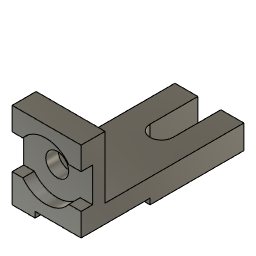
Tutorial Part 12 v5 (Autodesk Fusion 360 design; units mm, degrees)
Autodesk Fusion 360 part; units mm, degrees
sketch "Sketch1" plane through (0, 0, 0) normal (0, 1, 0) x (1, 0, 0)
  line L0 (-35.1053, -42) -> (36.8947, -42)
  line L1 (36.8947, -42) -> (36.8947, 48)
  line L2 (36.8947, 48) -> (-35.1053, 48)
  line L3 (-35.1053, 48) -> (-35.1053, -42)
  point P0 (0.8947, 48)
  dimension "d3" = 90
  dimension "d4" = 72
  dimension "d7" = 48
  constraint horizontal L0
  constraint vertical L1
  constraint horizontal L2
  constraint vertical L3
  constraint midpoint L2 P0
  measures "d3" distance of L0.start L2.end
  measures "d4" distance of L1.end L2.end
  measures "d7" vertical distance of origin P0
extrude "Extrude1" add sketch "Sketch1" along normal blind 25
sketch "Sketch2" plane through (0, 0, 0) normal (0, -1, 0) x (1, 0, 0)
  line L0 (-35.1053, 42) -> (-35.1053, -48)
  line L1 (-35.1053, -48) -> (36.8947, -48)
  line L2 (36.8947, -48) -> (36.8947, 42)
  line L3 (36.8947, 42) -> (-35.1053, 42)
  line L4 (-35.1053, -18) -> (-24, -18)
  line L5 (24, -18) -> (36.8947, -18)
  line L6 (24, 18) -> (36.8947, 18)
  line L7 (-24, 18) -> (-35.1053, 18)
  arc A0 (-24, -18) -> (24, -18) centre (0, 0) ccw
  arc A1 (24, 18) -> (-24, 18) centre (0, 0) ccw
  dimension "d11" = 60
  dimension "d12" = 30
  dimension "d13" = 36
  constraint coincident A0.centre A1.centre
  constraint coincident L0 L4.start
  constraint perpendicular L0 L4
  constraint coincident L2 L5.end
  constraint perpendicular L2 L5
  constraint coincident L6.start A0
  constraint coincident L2 L6.end
  constraint perpendicular L2 L6
  constraint coincident L0 L7.end
  constraint perpendicular L0 L7
  constraint collinear L4 L5
  constraint collinear L6 L7
  constraint concentric A0 A1
  measures "d11" diameter of A0
  measures "d12" distance of L1 L4
  measures "d13" distance of L4 L7
extrude "Extrude2" cut sketch "Sketch2" against normal blind 12 contours L0 L2 L4 L5 L6 L7 A0 A1
sketch "Sketch3" plane through (0, 12, 0) normal (0, -1, 0) x (1, 0, 0)
  arc A0 (24, 18) -> (-24, 18) centre (0, 0) ccw
  line L0 (-24, 18) -> (-35.1053, 18)
  line L1 (-35.1053, 18) -> (-35.1053, -18)
  line L2 (-35.1053, -18) -> (-24, -18)
  arc A1 (-24, -18) -> (24, -18) centre (0, 0) ccw
  line L3 (24, -18) -> (36.8947, -18)
  line L4 (36.8947, -18) -> (36.8947, 18)
  line L5 (36.8947, 18) -> (24, 18)
  circle A2 centre (0, 0) radius 12
  dimension "d16" = 24
  constraint concentric A0 A2
  measures "d16" diameter of A2
extrude "Extrude3" cut sketch "Sketch3" against normal blind 13 contours A2
sketch "Sketch4" plane through (0, 25, 0) normal (0, 1, 0) x (-1, 0, 0)
  circle A0 centre (0, 0) radius 12
  line L0 (35.1053, -48) -> (35.1053, 42)
  line L1 (35.1053, 42) -> (-36.8947, 42)
  line L2 (-36.8947, 42) -> (-36.8947, -48)
  line L3 (-36.8947, -48) -> (35.1053, -48)
  line L4 (-36.8947, -48) -> (35.1053, -48)
  line L5 (35.1053, -48) -> (35.1053, -23)
  line L6 (35.1053, -23) -> (-36.8947, -23)
  line L7 (-36.8947, -23) -> (-36.8947, -48)
  dimension "d19" = 25
  constraint horizontal L4
  constraint vertical L5
  constraint horizontal L6
  constraint vertical L7
  constraint coincident L0 L5.end
  constraint coincident L2.end L3.start
  measures "d19" distance of L0.start L5.end
extrude "Extrude4" add sketch "Sketch4" along normal blind 145 contours L0 L2 L3 L4 L5 L6 L7
sketch "Sketch5" plane through (0, 0, -23) normal (0, 0, 1) x (-1, 0, 0)
  line L0 (35.1053, -25) -> (-36.8947, -25)
  line L1 (-36.8947, -25) -> (-36.8947, -170)
  line L2 (-36.8947, -170) -> (35.1053, -170)
  line L3 (35.1053, -170) -> (35.1053, -25)
  line L4 (11.1053, -170) -> (11.1053, -120)
  arc A0 (11.1053, -120) -> (-12.8947, -120) centre (-0.8947, -120) ccw
  line L5 (-12.8947, -120) -> (-12.8947, -170)
  line L6 (11.1053, -170) -> (-12.8947, -170)
  dimension "d22" = 24
  dimension "d23" = 24
  dimension "d24" = 50
  constraint coincident L2 L4.start
  constraint perpendicular L2 L4
  constraint tangent L4 A0
  constraint coincident L2 L5.end
  constraint tangent A0 L5
  constraint perpendicular L2 L5
  measures "d22" distance of L1 L5
  measures "d23" distance of L4 L5
  measures "d24" distance of A0.end L5.end
extrude "Extrude5" cut sketch "Sketch5" against normal blind 25 contours L2 L4 A0 L5 L6
sketch "Sketch6" plane through (0, 0, -48) normal (0, 0, -1) x (1, 0, 0)
  line L0 (-11.1053, -170) -> (-11.1053, -120)
  arc A0 (12.8947, -120) -> (-11.1053, -120) centre (0.8947, -120) ccw
  line L1 (12.8947, -120) -> (12.8947, -170)
  line L2 (12.8947, -170) -> (36.8947, -170)
  line L3 (36.8947, -170) -> (36.8947, 0)
  line L4 (36.8947, 0) -> (-35.1053, 0)
  line L5 (-35.1053, 0) -> (-35.1053, -170)
  line L6 (-35.1053, -170) -> (-11.1053, -170)
  line L7 (36.8947, 0) -> (-11.1053, 0)
  line L8 (-11.1053, 0) -> (-11.1053, -72)
  line L9 (-11.1053, -72) -> (36.8947, -72)
  line L10 (36.8947, -72) -> (36.8947, 0)
  dimension "d27" = 48
  dimension "d28" = 72
  constraint horizontal L7
  constraint vertical L8
  constraint horizontal L9
  constraint vertical L10
  constraint coincident L3.end L4.start
  measures "d27" distance of L8.end L9.end
  measures "d28" distance of L7.end L8.end
extrude "Extrude6" cut sketch "Sketch6" against normal blind 6 contours L3 L4 L7 L8 L9 L10
